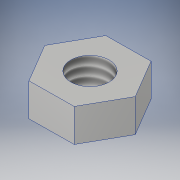
# Autodesk Inventor part: nut for base
Saved by Autodesk Inventor 2018 (Build 220112000, 112)
## iProperties
Created: 2018-03-02
Part Number: nut for base
Material: Aluminum 6061
Document SubType Name: Modeling
Designer: 238438
Density: 2.7 g/cm^3
Appearance: Aluminum - Flat
Mass: 0.248924 g
Surface Area: 1.63474 cm^2
Volume: 0.0921942 cm^3
Author: 238438
Autodesk Inventor part; units mm, degrees
ref_plane "YZ Plane" through (0, 0, 0) normal (1, 0, 0) x (0, 1, 0)
ref_plane "XZ Plane" through (0, 0, 0) normal (0, 1, 0) x (-1, 0, 0)
ref_plane "XY Plane" through (0, 0, 0) normal (0, 0, 1) x (1, 0, 0)
sketch "Sketch1" plane through (0, 0, 0) normal (0, 1, 0) x (-1, 0, 0)
  line L0 (1.945, 3.4488) -> (3.9593, 0.04)
  line L1 (3.9593, 0.04) -> (2.0143, -3.4088)
  line L2 (2.0143, -3.4088) -> (-1.945, -3.4488)
  line L3 (-1.945, -3.4488) -> (-3.9593, -0.04)
  line L4 (-3.9593, -0.04) -> (-2.0143, 3.4088)
  line L5 (-2.0143, 3.4088) -> (1.945, 3.4488)
  circle A0 centre (0, 0) radius 1.6955
  dimension "d0" = 6.858
  dimension "d1" = 3.3909
  constraints: 12 end point, 2 coincident, 1 centre point, 13 other
  measures "d0" distance between parallel lines of L2 L5
  measures "d1" diameter of A0
extrude "Extrusion1" add sketch "Sketch1" along normal blind 2.9083
thread "Thread1" size "8-32 UNC" class "2B" standard "ANSI Unified Screw Threads" full length
body "Solid1"
